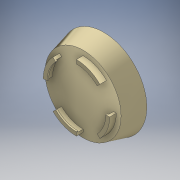
# Autodesk Inventor part: ET4
Saved by Autodesk Inventor 2016 (Build 200138000, 138)
## iProperties
Created: 2016-03-19
Part Number: ET4
Material: Genérico
Document SubType Name: Modeling
Designer: Usuario1
Density: 1 g/cm^3
Appearance: Valor por defecto
Author: Usuario1
Autodesk Inventor part; units mm, degrees
ref_plane "YZ Plane" through (0, 0, 0) normal (1, 0, 0) x (0, 1, 0)
ref_plane "XZ Plane" through (0, 0, 0) normal (0, 1, 0) x (-1, 0, 0)
ref_plane "XY Plane" through (0, 0, 0) normal (0, 0, 1) x (1, 0, 0)
sketch "Boceto1" plane through (0, 0, 0) normal (0, 0, 1) x (1, 0, 0)
  line L0 (-2.1248, 0.9275) -> (-1.8877, 0)
  line L1 (1.8773, 0) -> (2.1791, 0.9275)
  line L2 (2.1791, 0.9275) -> (-2.1248, 0.9275)
  line L3 (-1.8877, 0) -> (1.8773, 0)
  line L4 (-1.7761, 0.15) -> (1.7761, 0.15)
  line L5 (-1.9748, 0.9275) -> (-1.7761, 0.15)
  line L6 (1.7761, 0.15) -> (2.0291, 0.9275)
  line L7 (-2.1248, 0.9275) -> (-1.9748, 0.9275)
  line L8 (2.0291, 0.9275) -> (2.1791, 0.9275)
  line L9 (0, 0.15) -> (0, 0)
  line L10 (0, 0.15) -> (-1.7761, 0.15)
  line L11 (-1.8877, 0) -> (0, 0)
  constraints: 24 end point, 3 point on line, 1 midpoint
revolve "Revolución1" add sketch "Boceto1" angle 360 about axis through (0, 0.15, 0) along (0, -1, 0) contours L2 L5 L4 L9 L3 L0
sketch "Boceto2" plane through (0, 0.9275, 0) normal (0, 1, 0) x (1, 0, 0)
  circle A0 centre (0, 0) radius 2.1519
  circle A1 centre (0, 0) radius 2.0019
  line L0 (-1.9919, 0.2) -> (-1.6882, 0.2)
  line L1 (1.6882, 0.2) -> (1.9919, 0.2)
  line L2 (-1.9919, -0.2) -> (-1.6882, -0.2)
  line L3 (1.6882, -0.2) -> (1.9919, -0.2)
  line L4 (-0.2, -1.9919) -> (-0.2, -1.6882)
  line L5 (-0.2, 1.6882) -> (-0.2, 1.9919)
  line L6 (0.2, -1.9919) -> (0.2, -1.6882)
  line L7 (0.2, 1.6882) -> (0.2, 1.9919)
  arc A2 (0.2, 1.6882) -> (-0.2, 1.6882) centre (0, 0) ccw
  arc A3 (-1.6882, 0.2) -> (-1.6882, -0.2) centre (0, 0) ccw
  arc A4 (-0.2, -1.6882) -> (0.2, -1.6882) centre (0, 0) ccw
  arc A5 (1.6882, -0.2) -> (1.6882, 0.2) centre (0, 0) ccw
  constraints: 16 end point, 8 point on circle, 5 centre point, 10 other
extrude "Extrusión1" add sketch "Boceto2" against normal up to next contours A1 L3 A5 L1 | L7 A2 L5 A1 | A1 L4 A4 L6 | L0 A3 L2 A1
sketch "Boceto3" plane through (0, 0, 0) normal (0, -1, 0) x (1, 0, 0)
  arc A0 (1.0607, 1.0607) -> (0, 1.5) centre (0, 0) ccw
  arc A1 (0.9723, 0.9723) -> (0, 1.375) centre (0, 0) ccw
  arc A2 (1.0607, -1.0607) -> (1.5, 0) centre (0, 0) ccw
  arc A3 (0.9723, -0.9723) -> (1.375, 0) centre (0, 0) ccw
  arc A4 (-0.9723, -0.9723) -> (0, -1.375) centre (0, 0) ccw
  arc A5 (-1.0607, -1.0607) -> (0, -1.5) centre (0, 0) ccw
  arc A6 (-1.0607, 1.0607) -> (-1.5, 0) centre (0, 0) ccw
  arc A7 (-0.9723, 0.9723) -> (-1.375, 0) centre (0, 0) ccw
  arc A8 (0.9723, 0.9723) -> (0, 1.375) centre (0, 0) ccw
  line L0 (1.0607, 1.0607) -> (0.9723, 0.9723)
  line L1 (0, -1.5) -> (0, -1.375)
  line L2 (-0.9723, -0.9723) -> (-1.0607, -1.0607)
  line L3 (1.0607, -1.0607) -> (0.9723, -0.9723)
  line L4 (-0.9723, 0.9723) -> (-1.0607, 1.0607)
  line L5 (-1.5, 0) -> (-1.375, 0)
  line L6 (1.5, 0) -> (1.375, 0)
  line L7 (0, 1.5) -> (0, 1.375)
  line L8 (1.375, 0) -> (1.5, 0)
  line L9 (0.9723, -0.9723) -> (1.0607, -1.0607)
  arc A9 (0.9723, -0.9723) -> (1.375, 0) centre (0, 0) ccw
  arc A10 (1.0607, -1.0607) -> (1.5, 0) centre (0, 0) ccw
  point P0 (0, 0)
  constraints: 22 point on circle, 20 end point, 11 centre point, 2 collinear, 2 concentric, 2 horizontal, 2 perpendicular, 1 vertical
extrude "Extrusión2" add sketch "Boceto3" along normal blind 0.3
sketch "Boceto4" plane through (0, -0.3, 0) normal (0, -1, 0) x (1, 0, 0)
  arc A0 (0.9723, -0.9723) -> (1.375, 0) centre (0, 0) ccw projected
  arc A1 (0.9723, 0.9723) -> (0, 1.375) centre (0, 0) ccw projected
  arc A2 (-0.9723, 0.9723) -> (-1.375, 0) centre (0, 0) ccw projected
  arc A3 (-0.9723, -0.9723) -> (0, -1.375) centre (0, 0) ccw projected
  arc A4 (0.9369, -0.9369) -> (1.325, 0) centre (0, 0) ccw
  arc A5 (-0.9369, -0.9369) -> (0, -1.325) centre (0, 0) ccw
  arc A6 (0.9369, 0.9369) -> (0, 1.325) centre (0, 0) ccw
  arc A7 (-0.9369, 0.9369) -> (-1.325, 0) centre (0, 0) ccw
  line L0 (-0.9723, 0.9723) -> (-0.9369, 0.9369)
  arc A8 (-0.9723, 0.9723) -> (-1.375, 0) centre (0, 0) ccw projected
  line L1 (-1.375, 0) -> (-1.325, 0)
  arc A9 (-0.9723, -0.9723) -> (0, -1.375) centre (0, 0) ccw projected
  line L2 (-0.9369, -0.9369) -> (-0.9723, -0.9723)
  line L3 (0, 1.375) -> (0, 1.325)
  line L4 (0, -1.375) -> (0, -1.325)
  line L5 (0.9723, 0.9723) -> (0.9369, 0.9369)
  line L6 (1.375, 0) -> (1.325, 0)
  line L7 (0.9723, -0.9723) -> (0.9369, -0.9369)
  point P0 (0, 0)
  dimension "d7" = 0.05
  dimension "d8" = 0.05
  dimension "d9" = 0.05
  dimension "d10" = 0.05
  constraints: 16 end point, 8 point on circle, 4 centre point, 3 perpendicular, 1 collinear, 1 horizontal, 1 vertical
  measures "d7" radial gap between concentric circles of A0 A4
  measures "d8" radial gap between concentric circles of A3 A5
  measures "d9" radial gap between concentric circles of A1 A6
  measures "d10" radial gap between concentric circles of A2 A7
extrude "Extrusión3" add sketch "Boceto4" against normal blind 0.07
sketch "Boceto6" plane through (0, 0, 0) normal (0, 0, 1) x (1, 0, 0)
  spline S0 degree 2 poles (1.9646, 0.9275) (1.8594, 0.5179) (1.7648, 0.15) knots 0 0 0 1 1 1 weights 1 1.001423 1 projected
  line L0 (1.9646, 0.9275) -> (1.8046, 0.9275)
  line L1 (1.9646, 0.9275) -> (0.2, 0.9275) projected
  line L2 (1.7648, 0.15) -> (1.6048, 0.15)
  line L3 (1.7648, 0.15) -> (0.2, 0.15) projected
  line L4 (1.6048, 0.15) -> (1.8046, 0.9275)
  line L5 (0, 0) -> (0, 1.1488)
  dimension "d13" = 0.16
  dimension "d14" = 0.16
  constraints: 8 end point, 2 point on line, 1 vertical, 1 other
  measures "d13" distance of L0.start L0.end
  measures "d14" distance of L2.start L2.end
revolve "Revolución2" add sketch "Boceto6" angle 360 about axis through (0, 0, 0) along (0, 1, 0)
sketch "Boceto7" plane through (0, 0, 0) normal (0, 0, 1) x (1, 0, 0)
  line L0 (0.2, 0.15) -> (0.2, 0.9275) projected
  line L1 (1.7534, 0.15) -> (0.2, 0.15) projected
  spline S0 degree 4 poles (1.9544, 0.9275) (1.9026, 0.7268) (1.8518, 0.5303) (1.8021, 0.338) (1.7534, 0.15) knots 0 0 0 0 0 1 1 1 1 1 projected
  line L2 (1.9544, 0.9275) -> (1.9544, 0.9275) projected
  line L3 (1.7648, 0.15) -> (1.7534, 0.15) projected
  line L4 (1.9544, 0.9275) -> (1.7534, 0.15)
  line L5 (1.8877, 0) -> (2.1248, 0.9275) projected
  line L6 (2.1248, 0.9275) -> (-2.1248, 0.9275) projected
  line L7 (1.8877, 0) -> (-1.8877, 0) projected
  line L8 (2.1248, 0.9275) -> (-2.1248, 0.9275) projected
  line L9 (1.8877, 0) -> (-1.8877, 0) projected
  line L10 (2.1248, 0.9275) -> (1.8877, 0)
  line L11 (1.8877, 0) -> (1.7174, 0)
  line L12 (1.7174, 0) -> (1.9544, 0.9275)
  line L13 (2.1248, 0.9275) -> (1.9544, 0.9275)
  line L14 (1.9646, 0.9275) -> (1.9544, 0.9275) projected
  line L15 (0, 0) -> (0.9723, 0) projected
  line L16 (0, 0) -> (0, 1.1666)
  constraints: 12 end point, 2 collinear, 1 parallel, 1 point on line, 1 vertical, 1 other
revolve "Revolución3" cut sketch "Boceto7" angle 360 about axis through (0, 0, 0) along (0, 1, 0) contours L6 L5 L7 L12
